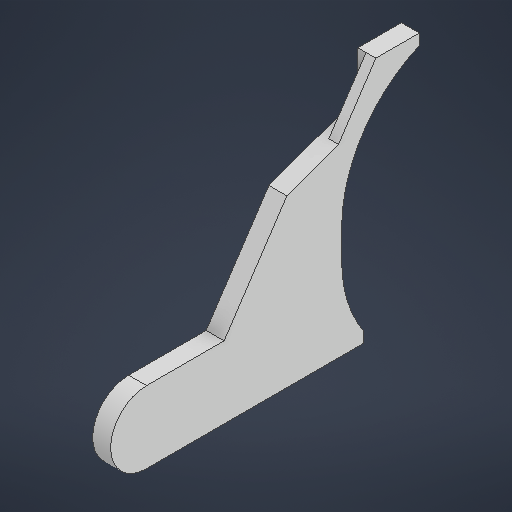
# Autodesk Inventor part: body-main
Saved by Autodesk Inventor 2025 (Build 290162000, 162)
## iProperties
Created: 2025-03-21
Part Number: body-main
Material: Všeobecné
Document SubType Name: Modeling
Designer: Simak
Density: 1 g/cm^3
Appearance: Výchozí
Author: Simak
Autodesk Inventor part; units mm, degrees
ref_plane "YZ Plane" through (0, 0, 0) normal (1, 0, 0) x (0, 1, 0)
ref_plane "XZ Plane" through (0, 0, 0) normal (0, 1, 0) x (-1, 0, 0)
ref_plane "XY Plane" through (0, 0, 0) normal (0, 0, 1) x (1, 0, 0)
sketch "Náčrt1" plane through (0, 0, 0) normal (1, 0, 0) x (0, 1, 0)
  circle A0 centre (13.5, 0) radius 16.5 construction
  circle A1 centre (15.5, 0) radius 16.5 construction
  circle A2 centre (11.5, 0) radius 16.5 construction
  line L0 (15.5, 16.5) -> (11.5, 16.5) construction
  line L1 (15.5, -16.5) -> (11.5, -16.5) construction
  circle A3 centre (5, 45.139) radius 5
  line L2 (0, 0) -> (0, 45.139)
  line L3 (10, 34.353) -> (23.0973, 25.6215)
  line L4 (10, 34.353) -> (10, 45.139)
  line L5 (23.0973, 25.6215) -> (27.6, 13.25)
  line L6 (27.6, 13.25) -> (33.5, 13.25)
  line L7 (33.5, 13.25) -> (25.7098, 18.4434)
  line L8 (33.5, 13.25) -> (33.5, 7.1937)
  line L9 (29.1, 13.25) -> (27.1194, 14.5704)
  arc A4 (13.5, -17.8885) -> (15.5, 18) centre (15.5, 0) ccw
  arc A5 (11.5, 18) -> (13.5, -17.8885) centre (11.5, 0) ccw
  line L10 (15.5, 18) -> (11.5, 18)
  line L11 (1.5, 14.9666) -> (0, 14.9666)
  line L12 (33.5, 7.1937) -> (32, 7.1937)
  arc A6 (13.5, -19.4977) -> (15.5, 19.6) centre (15.5, 0) ccw
  arc A7 (11.5, 19.6) -> (13.5, -19.4977) centre (11.5, 0) ccw
  line L13 (11.5, 19.6) -> (15.5, 19.6)
  line L14 (21, 28.6) -> (0, 28.6) construction
  line L15 (0, 28.6) -> (0, 19.6)
  line L16 (0, 19.6) -> (21, 19.6)
  line L17 (21, 19.6) -> (21, 28.6) construction
  line L18 (35.6, 21.5) -> (34, 21.5) construction
  line L19 (34, 21.5) -> (34, -16) construction
  line L20 (34, -16) -> (35.6, -16) construction
  line L21 (35.6, -16) -> (35.6, 21.5) construction
  line L22 (35.6, 17.75) -> (34, 17.75) construction
  line L23 (33.2196, 14.55) -> (26.5242, 14.55) construction
  point P0 (26.5242, 16.2057)
  dimension "d0" = 33
  dimension "d1" = 2
  dimension "d2" = 2
  dimension "d3" = 13.5
  dimension "d4" = 10
  dimension "d5" = 45.139
  dimension "d6" = 10.786
  dimension "d8" = 123.69
  dimension "d9" = 15.741
  dimension "d10" = 13.25
  dimension "d11" = 33.5
  dimension "d12" = 5.9
  dimension "d16" = 1.5
  dimension "d17" = 36
  dimension "d18" = 36
  dimension "d19" = 1.5
  dimension "d20" = 1.5
  dimension "d21" = 1.6
  dimension "d23" = 9
  dimension "d24" = 21
  dimension "d25" = 0.5
  dimension "d26" = 1.6
  dimension "d27" = 37.5
  dimension "d28" = 3.75
  dimension "d29" = 20.5
  dimension "d30" = 3.2
  constraints: 48 end point, 17 point on circle, 8 centre point, 8 point on line, 7 horizontal, 6 perpendicular, 5 parallel, 5 tangent, 3 horizontal alignment, 3 vertical, 2 coincident, 2 equal radius, 1 collinear, 2 other
  measures "d0" diameter of A0
  measures "d1" distance of A0.centre A1.centre
  measures "d2" distance of A0.centre A2.centre
  measures "d3" distance of A0.centre L2.start
  measures "d4" diameter of A3
  measures "d5" vertical distance of A3.centre A0.centre
  measures "d6" vertical distance of A3.centre L3.start
  measures "d8" angle of L4 L3
  measures "d9" distance of L3.start L3.end
  measures "d10" distance from line of A1.centre L6
  measures "d11" distance from line of L2 L6.end
  measures "d12" distance of L5.end L6.end
  measures "d16" distance of L5.end L9.start
  measures "d17" diameter of A4
  measures "d18" diameter of A5
  measures "d19" distance of L11.start L11.end
  measures "d20" distance of L8.end L12.end
  measures "d21" radial gap between concentric circles of A4 A6
  measures "d23" distance of L16.end L14.start
  measures "d24" distance of L14.start L14.end
  measures "d25" distance between parallel lines of L20 L1
  measures "d26" distance of L19.end L20.end
  measures "d27" distance of L20.end L18.start
  measures "d28" distance between parallel lines of L18 L22
  measures "d29" distance from line of L19 A0.centre
  measures "d30" distance between parallel lines of L22 L23
extrude "Vysunutí1" add sketch "Náčrt1" against normal blind 2.5 contours A3 | L4 L3 L5 A6 L13 L16 L2 A3 | L16 A7 L2 | A7 L13 A6 L5 A4 L10 A5 L11 L2 | L8 A6 L6 | L9 L6 A4 L5 | A6 L8 L12 A4 L6
extrude "Vysunutí2" add sketch "Náčrt1" against normal blind 1.35 contours L7 L6 A6 L5 | A6 L6 L9 L5
equation "\"d2\" = d1"
equation "\"d18\" = d17"
